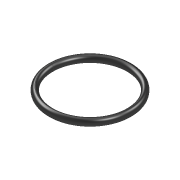
# Autodesk Inventor part: Junta_torica_pieza_sonar
Saved by Autodesk Inventor 2022.3 (Build 263350000, 350)
## iProperties
Created: 2023-07-17
Part Number: Junta_torica_pieza_sonar
Material: Genérico
Document SubType Name: Modeling
Designer: Usuario
Density: 1 g/cm^3
Appearance: Valor por defecto
Author: Usuario
Autodesk Inventor part; units mm, degrees
ref_plane "YZ Plane" through (0, 0, 0) normal (1, 0, 0) x (0, 1, 0)
ref_plane "XZ Plane" through (0, 0, 0) normal (0, 1, 0) x (-1, 0, 0)
ref_plane "XY Plane" through (0, 0, 0) normal (0, 0, 1) x (1, 0, 0)
sketch "Boceto1" plane through (0, 0, 0) normal (1, 0, 0) x (0, 1, 0)
  line L0 (0, 0) -> (2, 0)
  line L1 (0, 0) -> (0, -1.65)
  ellipse E0 centre (0, 0) end of major axis (2, 0) minor radius 1.65
  dimension "d0" = 2
  dimension "d1" = 1.65
  constraints: 4 end point, 2 horizontal, 1 coincident, 1 vertical, 4 other
  measures "d0" distance of L0.start L0.end
  measures "d1" distance of L0.start L1.end
sketch "Boceto2" plane through (0, 0, 0) normal (0, 1, 0) x (-1, 0, 0)
  line L0 (0, 0) -> (0, -21.75)
  circle A0 centre (0, -21.75) radius 21.75
  dimension "d2" = 21.75
  constraints: 2 end point, 1 coincident, 1 vertical, 1 vertical alignment, 2 other
  measures "d2" distance of L0.start L0.end
sweep "Barrido1" add profiles "Boceto1" path "Boceto2" path curves A0
